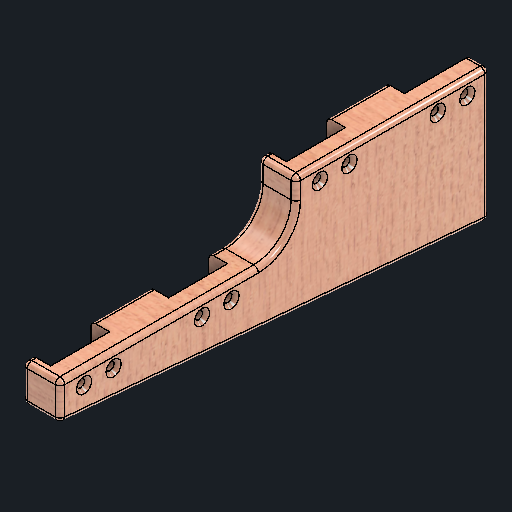
# Autodesk Inventor part: Side
Saved by Autodesk Inventor 2026.2 (Build 302298000, 298)
## iProperties
Created: 2026-10-05
Part Number: Side
Material: Wood (Oak)
Document SubType Name: Modeling
Designer: JoshuaEah
Density: 0.76 g/cm^3
Appearance: White Oak - Natural Medium Gloss
Author: JoshuaEah
Revision Number: 2
Autodesk Inventor part; units mm, degrees
ref_plane "YZ Plane" through (0, 0, 0) normal (1, 0, 0) x (0, 1, 0)
ref_plane "XZ Plane" through (0, 0, 0) normal (0, 1, 0) x (-1, 0, 0)
ref_plane "XY Plane" through (0, 0, 0) normal (0, 0, 1) x (1, 0, 0)
sketch "Sketch1" plane through (0, 0, 0) normal (1, 0, 0) x (0, 1, 0)
  line L0 (0, 0) -> (20, 0)
  line L1 (20, 0) -> (20, -46.35)
  line L2 (20, -46.35) -> (0, -46.35)
  line L3 (0, -46.35) -> (0, 0)
  line L4 (0, -86.35) -> (20, -86.35)
  line L5 (20, -86.35) -> (20, -126.35)
  line L6 (20, -126.35) -> (0, -126.35)
  line L7 (0, -126.35) -> (0, -86.35)
  line L8 (40, -246.35) -> (60, -246.35)
  line L9 (60, -286.35) -> (40, -286.35)
  line L10 (40, -286.35) -> (40, -246.35)
  line L11 (-5, 0) -> (20, 0)
  line L12 (20, 0) -> (20, -160)
  line L13 (20, -160) -> (60, -160)
  line L14 (60, -160) -> (60, -291.35)
  line L15 (60, -291.35) -> (-30.5, -291.35)
  line L16 (-5, 0) -> (-30.5, -291.35)
  line L17 (-5, 0) -> (-5, -291.35)
  line L18 (40, -286.35) -> (-30.0624, -286.35)
  line L19 (60, -206.35) -> (40, -206.35)
  line L20 (40, -206.35) -> (40, -166.35)
  line L21 (40, -166.35) -> (60, -166.35)
  line L22 (20, -6.35) -> (0, -6.35)
  point P0 (10, -16.35)
  point P1 (50, -176.35)
  point P2 (10, -36.35)
  point P3 (10, -96.35)
  point P4 (10, -116.35)
  point P5 (50, -196.35)
  point P6 (50, -256.35)
  point P7 (50, -276.35)
  point P8 (20, -46.35)
  point P9 (57.9398, -280.8611)
  point P10 (57.9398, -240.8611)
  point P11 (20, -86.35)
  point P12 (-39.3797, -280)
  point P13 (10, -6.35)
  point P14 (50, -166.35)
  dimension "d0" = 20
  dimension "d3" = 40
  dimension "d4" = 40
  dimension "d19" = 5
  dimension "d52" = 5
  dimension "d60" = 90.5
  dimension "d66" = 6.35
  dimension "d67" = 20
  dimension "d68" = 40
  dimension "d69" = 40
  dimension "d70" = 6.35
  dimension "d71" = 40
  dimension "d72" = 10
  dimension "d73" = 10
  dimension "d74" = 10
  dimension "d75" = 10
  dimension "d76" = 10
  dimension "d77" = 10
  dimension "d78" = 10
  dimension "d79" = 10
  dimension "d80" = 40
  dimension "d81" = 20
  dimension "d82" = 40
  constraints: 46 end point, 10 perpendicular, 10 point on line, 8 vertical alignment, 6 horizontal, 5 parallel, 3 collinear, 2 midpoint, 1 coincident
  measures "d0" distance of L1.end L2.end
  measures "d3" distance of L4.end L5.end
  measures "d4" distance between parallel lines of L2 L4
  measures "d19" distance between parallel lines of L9 L15
  measures "d52" distance between parallel lines of L7 L17
  measures "d60" distance of L14.end L15.end
  measures "d66" distance between parallel lines of L21 L13
  measures "d67" distance of L19.start L19.end
  measures "d68" distance between parallel lines of L6 L21
  measures "d69" distance of L19.end L20.end
  measures "d70" distance between parallel lines of L11 L22
  measures "d71" distance between parallel lines of L22 L2
  measures "d72" distance from line of L22 point (10, -16.35)
  measures "d73" distance from line of L2 point (10, -36.35)
  measures "d74" distance from line of L4 point (10, -96.35)
  measures "d75" distance from line of L6 point (10, -116.35)
  measures "d76" distance from line of point (50, -176.35) L21
  measures "d77" distance from line of point (50, -196.35) L19
  measures "d78" distance from line of point (50, -256.35) L8
  measures "d79" distance from line of L9 point (50, -276.35)
  measures "d80" distance of L9.end L8.start
  measures "d81" distance between parallel lines of L12 L20
  measures "d82" distance between parallel lines of L19 L8
extrude "Extrusion1" add sketch "Sketch1" against normal blind 12.7
extrude "Extrusion2" add sketch "Sketch1" against normal blind 12.7 from surface at -12.7 contours L0 L1 L22 L3 | L3 L2 L12 L4 L7 L6 L13 L14 L21 L20 L19 L8 L10 L18 L17 L11 | L17 L18 L16
fillet "Rounded Features" radius 3.175 5 edges at (-12.7, 20, 0) (-12.7, 60, -160) (-6.35, 60, -291.35) (-6.35, -30.5, -291.35) (-12.7, -5, 0)
fillet "Rounded Features" radius 25.4 1 edges at (-12.7, 20, -160)
fillet "Outside Edgebreak" radius 3.175 12 edges at (0, 59.0701, -160.9299) (0, 51.1125, -160) (0, 27.4395, -152.5605) (0, 20, -68.8875) (0, 19.0701, -0.9299) (0, 7.3671, 0) (0, -4.2357, -0.8341) (0, -17.7258, -145.3982) (0, -29.3759, -290.32) (0, 14.895, -291.35) (0, 59.0701, -290.4201) (0, 60, -225.675)
fillet "Internal Edgebreak" radius 3.175 12 edges at (-25.4, 20, -130.475) (-25.4, 51.1125, -160) (-25.4, 59.0701, -160.9299) (-25.4, 60, -164.7625) (-25.4, 27.4395, -152.5605) (-25.4, -4.2357, -0.8341) (-25.4, -17.658, -144.6241) (-25.4, 19.0701, -0.9299) (-25.4, 20, -4.7625) (-25.4, 7.3671, 0) (-25.4, 20, -66.35) (-25.4, 60, -226.35)
fillet "Shelf Edgebreak" radius 0.4 8 edges at (-19.05, 40, -246.35) (-19.05, 40, -286.35) (-19.05, 40, -206.35) (-19.05, 40, -166.35) (-19.05, 0, -126.35) (-19.05, 0, -86.35) (-19.05, 0, -46.35) (-19.05, 0, -6.35)
hole "Hole1" at (0, 10, -16.35) direction (-1, 0, 0) diameter 5.5118 end through all start extended yes countersink diameter 10.3886 countersink angle 90 clearance for "Flat Head Machine Screw" size "M5" standard "Ansi Metric M Profile"
pattern_sketch "Sketch Driven Pattern1" of "Hole1" from (0, 10, -16.35) copies at (0, 50, -176.35) at (0, 10, -36.35) at (0, 10, -96.35) at (0, 10, -116.35) at (0, 50, -196.35) at (0, 50, -256.35) at (0, 50, -276.35)
body "Solid1"
